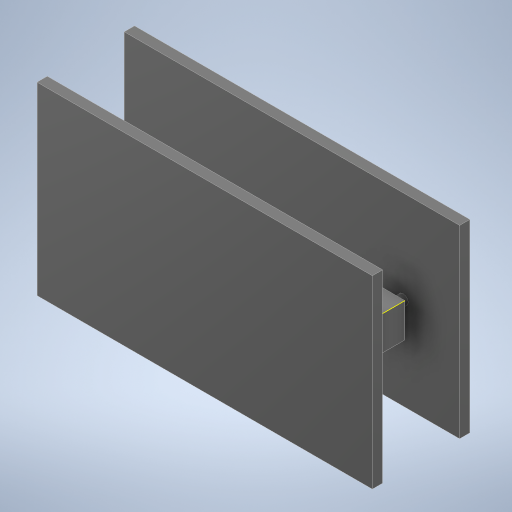
# Autodesk Inventor part: load_cell
Saved by Autodesk Inventor 2023 (Build 270158000, 158)
## iProperties
Created: 2023-03-09
Part Number: load_cell
Material: Acetal Resin, Black
Document SubType Name: Modeling
Designer: Amanda Fontes
Density: 1.425 g/cm^3
Appearance: Smooth - Black
Author: Amanda Fontes
Autodesk Inventor part; units mm, degrees
ref_plane "YZ Plane" through (0, 0, 0) normal (1, 0, 0) x (0, 1, 0)
ref_plane "XZ Plane" through (0, 0, 0) normal (0, 1, 0) x (-1, 0, 0)
ref_plane "XY Plane" through (0, 0, 0) normal (0, 0, 1) x (1, 0, 0)
sketch "loadcell" plane through (0, 0, 0) normal (0, 1, 0) x (-1, 0, 0)
  line L0 (0, 0) -> (76, 0)
  line L1 (76, 0) -> (76, -12.5)
  line L2 (76, -12.5) -> (0, -12.5)
  line L3 (0, -12.5) -> (0, 0)
  point P0 (38, -6.25)
  dimension "d0" = 76
  dimension "d1" = 12.5
  constraints: 8 end point, 2 parallel, 1 horizontal, 1 perpendicular
  measures "d0" distance of L1.end L2.end
  measures "d1" distance of L0.end L1.end
extrude "Base" add sketch "loadcell" along normal blind 10
sketch "Sketch3" plane through (0, 10, 0) normal (0, 1, 0) x (1, 0, 0)
  line L0 (-76, 12.5) -> (-76, 0) projected
  line L1 (-76, 6.25) -> (0, 6.25)
  line L2 (0, 12.5) -> (-76, 12.5) projected
  line L3 (-38, 12.5) -> (-38, 0)
  circle A0 centre (-36, 6.25) radius 4
  circle A1 centre (-40, 6.25) radius 4
  point P0 (0, 0)
  point P1 (-38, 6.25)
  point P2 (-38, 9.7141)
  point P3 (-38, 6.25)
  dimension "d4" = 8
  dimension "d5" = 8
  dimension "d8" = 2
  dimension "d9" = 2
  constraints: 4 end point, 4 midpoint, 2 centre point, 2 coincident, 2 point on line, 1 horizontal, 1 vertical
  measures "d4" diameter of A0
  measures "d5" diameter of A1
  measures "d8" distance from line of L3 A1.centre
  measures "d9" distance of point (-38, 6.25) A0.centre
extrude "Furo" cut sketch "Sketch3" against normal blind 10 contours A1 A0 L1 | L1 A0 A1 | A1 L1 L3 | L3 L1 A0 | A0 L1 A1 | L1 L3 A0 | A1 L1 A0 | L3 L1 A1
sketch "Sketch2" plane through (0, 10, 0) normal (0, 1, 0) x (1, 0, 0)
  line L0 (-76, 12.5) -> (-76, 0) projected
  line L1 (0, 0) -> (0, 12.5) projected
  point P0 (-38, 6.25)
sketch "Sketch4" plane through (-76, 0, 0) normal (0, 0, 1) x (1, 0, 0)
  line L0 (76, 0) -> (76, 10) projected
  line L1 (0, 0) -> (0, 10) projected
  line L2 (76, 10) -> (0, 10) projected
  line L3 (76, 0) -> (0, 0) projected
  line L4 (0, 0) -> (0, 10) projected
  line L5 (38, 10) -> (38, 0)
  point P0 (38, 5)
  point P1 (5.5, 5)
  point P2 (15.5, 5)
  point P3 (0, 5)
  point P4 (0, 5)
  point P5 (70.5, 5)
  point P6 (60.5, 5)
  dimension "d12" = 5.5
  dimension "d13" = 15.5
  constraints: 4 midpoint, 2 end point, 2 symmetric about line, 1 perpendicular
  measures "d12" distance of point (5.5, 5) point (0, 5)
  measures "d13" distance of point (15.5, 5) point (0, 5)
hole "Hole1" at (-70.5, 5, 0) at (-60.5, 5, 0) direction (0, 0, -1) diameter 3 end through all
thread "Thread1" size "M3x0.5" class "6H" standard "ANSI Metric M Profile" full length
thread "Thread2" size "M3x0.5" class "6H" standard "ANSI Metric M Profile" full length
thread "Thread3" size "M3x0.5" class "6H" standard "ANSI Metric M Profile" full length
hole "Hole2" at (-15.5, 5, 0) at (-5.5, 5, 0) direction (0, 0, -1) diameter 3 end through all
thread "Thread4" size "M3x0.5" class "6H" standard "ANSI Metric M Profile" full length
thread "Thread5" size "M3x0.5" class "6H" standard "ANSI Metric M Profile" full length
sketch "pino_de_baixo" plane through (-76, 0, 0) normal (0, 0, 1) x (1, 0, 0)
  circle A0 centre (5.5, 5) radius 1.5 projected
  circle A1 centre (5.5, 5) radius 1.5
  point P0 (76, 0)
  constraints: 1 centre point, 1 coincident
extrude "parafuso/pino" add sketch "pino_de_baixo" along normal blind 5
sketch "Sketch6" plane through (-70.5, 5, 5) normal (0, 0, 1) x (1, 0, 0)
  line L0 (-16.5, 27) -> (81.5, 27)
  line L1 (81.5, 27) -> (81.5, -27)
  line L2 (81.5, -27) -> (-16.5, -27)
  line L3 (-16.5, -27) -> (-16.5, 27)
  dimension "d48" = 98
  dimension "d49" = 54
  constraints: 8 end point, 2 parallel, 1 horizontal, 1 perpendicular
  measures "d48" distance of L0.start L0.end
  measures "d49" distance of L0.end L1.end
extrude "Extrusion4" add sketch "Sketch6" along normal blind 3
sketch "pino/furo/ima" plane through (0, 0, -12.5) normal (0, 0, -1) x (-1, 0, 0)
  circle A0 centre (5.5, 5) radius 1.5 projected
  circle A1 centre (5.5, 5) radius 1.5
  point P0 (0, 0)
  constraints: 1 centre point, 1 coincident
extrude "Extrusion5" add sketch "pino/furo/ima" along normal blind 5
sketch "Sketch8" plane through (-5.5, 5, -17.5) normal (0, 0, -1) x (-1, 0, 0)
  line L0 (81.5, -27) -> (-16.5, -27) projected
  line L1 (81.5, 27) -> (81.5, -27) projected
  line L2 (-16.5, -27) -> (81.5, -27)
  line L3 (81.5, -27) -> (81.5, 27)
  line L4 (81.5, 27) -> (-16.5, 27)
  line L5 (-16.5, 27) -> (-16.5, -27)
  point P0 (-5.5, -5)
  constraints: 8 end point, 2 parallel, 1 horizontal, 1 perpendicular
extrude "Extrusion6" add sketch "Sketch8" along normal blind 3
sketch "ima-neodimio" plane through (-5.5, 5, -20.5) normal (0, 0, -1) x (-1, 0, 0)
  line L0 (32.5, 5) -> (32.5, -5) projected
  arc A0 (12.0929, -3.2123) -> (33.5362, -3.1801) centre (22.8022, 5.0619) ccw construction
  arc A1 (-2.547, 2.3582) -> (24.0058, 2.3582) centre (10.7294, 12.6379) ccw
  arc A2 (2.6045, 6.3469) -> (18.8543, 6.3469) centre (10.7294, 12.6379) ccw
  arc A3 (2.6045, 6.3469) -> (-2.547, 2.3582) centre (0.0287, 4.3526) ccw
  arc A4 (24.0058, 2.3582) -> (18.8543, 6.3469) centre (21.4301, 4.3526) ccw
  arc A5 (56.7203, -3.2123) -> (78.1636, -3.1801) centre (67.4295, 5.0619) ccw construction
  arc A6 (42.0804, 2.3582) -> (68.6332, 2.3582) centre (55.3568, 12.6379) ccw
  arc A7 (47.2319, 6.3469) -> (63.4817, 6.3469) centre (55.3568, 12.6379) ccw
  arc A8 (47.2319, 6.3469) -> (42.0804, 2.3582) centre (44.6561, 4.3526) ccw
  arc A9 (68.6332, 2.3582) -> (63.4817, 6.3469) centre (66.0575, 4.3526) ccw
  constraints: 20 point on circle, 10 centre point, 8 tangent
extrude "Extrusion7" add sketch "ima-neodimio" along normal blind 1.5
